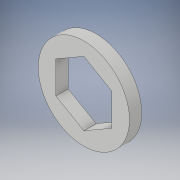
# Autodesk Inventor part: 2AM-17-P-7201 - sproket thing ig
Saved by Autodesk Inventor 2017 (Build 210142000, 142)
## iProperties
Created: 2017-12-28
Part Number: 2AM-17-P-7201 - sproket thing ig
Material: Generic
Document SubType Name: Modeling
Designer: Micah
Density: 1 g/cm^3
Appearance: Default
Author: Micah
Autodesk Inventor part; units mm, degrees
ref_plane "YZ Plane" through (0, 0, 0) normal (1, 0, 0) x (0, 1, 0)
ref_plane "XZ Plane" through (0, 0, 0) normal (0, 1, 0) x (-1, 0, 0)
ref_plane "XY Plane" through (0, 0, 0) normal (0, 0, 1) x (1, 0, 0)
sketch "Sketch1" plane through (0, 0, 0) normal (0, 0, 1) x (1, 0, 0)
  circle A0 centre (0, 0) radius 10.4013
  line L0 (0, 7.347) -> (6.3627, 3.6735)
  line L1 (6.3627, 3.6735) -> (6.3627, -3.6735)
  line L2 (6.3627, -3.6735) -> (0, -7.347)
  line L3 (-6.3627, -3.6735) -> (0, -7.347)
  line L4 (-6.3627, -3.6735) -> (-6.3627, 3.6735)
  line L5 (0, 7.347) -> (-6.3627, 3.6735)
  dimension "d0" = 20.8026
  constraints: 12 end point, 1 centre point, 1 coincident, 1 parallel
  measures "d0" diameter of A0
extrude "Extrusion1" add sketch "Sketch1" along normal blind 2.794
body "Solid1"
